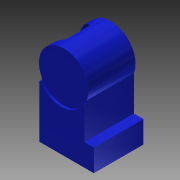
# Autodesk Inventor part: LEG RHS
Saved by Autodesk Inventor 2015 (Build 190159000, 159)
## iProperties
Created: 2012-05-01
Part Number: LEG RHS
Material: 250
Document SubType Name: Modeling
Mass: 3.79543 g
Surface Area: 5.29638 cm^2
Volume: 0.483494 cm^3
Density: 7.85 g/cm^3
Appearance: Steel
Autodesk Inventor part; units mm, degrees
ref_plane "YZ Plane" through (0, 0, 0) normal (1, 0, 0) x (0, 1, 0)
ref_plane "XZ Plane" through (0, 0, 0) normal (0, 1, 0) x (-1, 0, 0)
ref_plane "XY Plane" through (0, 0, 0) normal (0, 0, 1) x (1, 0, 0)
sketch "Sketch1" plane through (0, 0, 0) normal (0, 0, 1) x (1, 0, 0)
  line L0 (-3.154, -9.45) -> (4.676, -9.45)
  line L1 (4.676, -9.45) -> (4.676, -6.279)
  line L2 (4.676, -6.279) -> (3.303, -6.279)
  line L3 (3.303, -6.279) -> (3.303, -1.2735)
  line L4 (-3.154, -9.45) -> (-3.154, -1.6074)
  arc A0 (3.303, -1.2735) -> (-3.154, -1.6074) centre (0, 0) ccw
  dimension "d0" = 7.83
  dimension "d1" = 9.45
  dimension "d2" = 3.54
  dimension "d3" = 3.154
  dimension "d4" = 3.171
  dimension "d5" = 6.457
  constraints: 10 end point, 3 parallel, 2 point on circle, 1 centre point, 1 coincident, 1 horizontal, 1 perpendicular
  measures "d0" distance of L0.start L0.end
  measures "d1" distance from line of L0 point (0, 0)
  measures "d2" radius of A0
  measures "d3" distance from line of point (0, 0) L4
  measures "d4" distance of L0.end L1.end
  measures "d5" distance between parallel lines of L4 L3
extrude "Extrusion1" add sketch "Sketch1" along normal mid plane 7.108
sketch "Sketch2" plane through (-3.154, -9.45, 3.554) normal (0, -1, 0) x (1, 0, 0)
  line L0 (7.83, -7.108) -> (7.83, 0) projected
  circle A0 centre (4.63, -3.554) radius 2.5
  point P0 (3.154, -3.554)
  dimension "d8" = 5
  dimension "d9" = 3.2
  constraints: 1 centre point, 1 horizontal alignment
  measures "d8" diameter of A0
  measures "d9" distance from line of L0 A0.centre
extrude "Extrusion2" cut sketch "Sketch2" against normal blind 2
sketch "Sketch3" plane through (-3.154, -9.45, 3.554) normal (-1, 0, 0) x (0, 0, 1)
  line L0 (0, 0) -> (-7.108, 0) projected
  circle A0 centre (-3.554, 3) radius 2.5
  point P0 (-3.554, 9.45)
  dimension "d12" = 5
  dimension "d13" = 3
  constraints: 1 centre point, 1 vertical alignment
  measures "d12" diameter of A0
  measures "d13" distance from line of A0.centre L0
extrude "Extrusion3" cut sketch "Sketch3" against normal blind 2
sketch "Sketch4" plane through (-1.154, -6.45, 0) normal (-1, 0, 0) x (0, 0, 1)
  circle A0 centre (0, 0) radius 2.5 construction
  circle A1 centre (0, 8) radius 2.5
  circle A2 centre (0, 0) radius 2.5 projected
  point P0 (0, 6.45)
  dimension "d16" = 8
  constraints: 1 centre point, 1 equal radius, 1 vertical alignment
  measures "d16" distance of A0.centre A1.centre
extrude "Extrusion4" cut sketch "Sketch4" along normal through all contours A1
sketch "Sketch6" plane through (0, 0, 3.554) normal (0, 0, 1) x (1, 0, 0)
  arc A0 (3.303, -1.2735) -> (-3.154, -1.6074) centre (0, 0) ccw projected
  circle A1 centre (0, 0) radius 3.54
  constraints: 1 coincident, 3 other
extrude "Extrusion6" cut sketch "Sketch6" against normal blind 0.345
fillet "Fillet2" radius 0.1 2 edges at (-3.154, -1.6074, 3.3815) (3.303, -1.2735, 3.3815)
body "Solid1"
